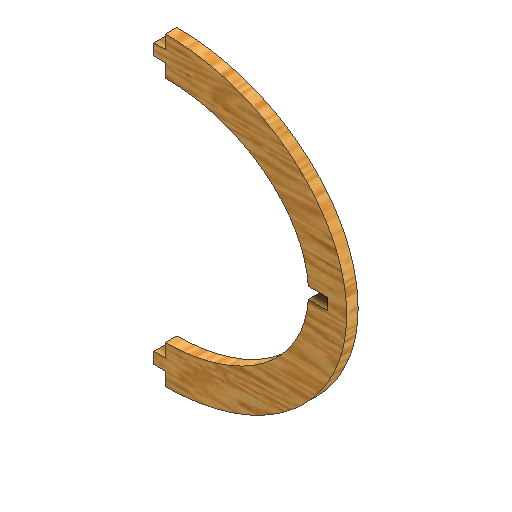
# Autodesk Inventor part: Arch Rear Outer
Saved by Autodesk Inventor 2025.2 (Build 292293000, 293)
## iProperties
Created: 2025-01-15
Part Number: Arch Rear Outer
Material: Plywood, Sheathing
Document SubType Name: Modeling
Designer: alexb
Density: 0.552 g/cm^3
Appearance: Plywood - New
Author: alexb
Autodesk Inventor part; units mm, degrees
ref_plane "YZ Plane" through (0, 0, 0) normal (1, 0, 0) x (0, 1, 0)
ref_plane "XZ Plane" through (0, 0, 0) normal (0, 1, 0) x (-1, 0, 0)
ref_plane "XY Plane" through (0, 0, 0) normal (0, 0, 1) x (1, 0, 0)
sketch "Sketch1" plane through (0, 0, 0) normal (0, 0, 1) x (1, 0, 0)
  ellipse E0 centre (0, 0) end of major axis (95, 0) minor radius 80 (0, -80) -> (0, 80) ccw
  ellipse E1 centre (0, 0) end of major axis (75, 0) minor radius 60 (0, -60) -> (0, 60) ccw
  line L0 (0, 80) -> (0, 73)
  line L1 (0, 73) -> (-6, 73)
  line L2 (-6, 73) -> (-6, 67)
  line L3 (-6, 67) -> (0, 67)
  line L4 (0, 67) -> (0, 60)
  line L5 (75, 0) -> (95, 0) construction
  line L6 (0, -73) -> (-6, -73)
  line L7 (-6, -73) -> (-6, -67)
  line L8 (-6, -67) -> (0, -67)
  line L9 (0, -60) -> (0, -67)
  line L10 (0, -73) -> (0, -80)
  line L11 (85, -35.7275) -> (85, 35.7275) construction
  line L12 (85, 3) -> (85, -3)
  line L13 (85, 3) -> (74.9062, 3)
  line L14 (85, -3) -> (74.9062, -3)
  point P0 (85, 0)
  dimension "d0" = 80
  dimension "d2" = 75
  dimension "d3" = 60
  dimension "d4" = 95
  dimension "d6" = 6
  dimension "d7" = 6
  constraints: 30 end point, 7 vertical, 5 perpendicular, 4 symmetric about line, 3 horizontal, 3 midpoint, 2 coincident, 2 equal length, 1 point on line, 13 other
  measures "d6" distance of L1.end L2.end
  measures "d7" distance between parallel lines of L14 L13
extrude "Extrusion1" add sketch "Sketch1" along normal blind 6 contours L10 L6 L7 L8 L9 E1 L14 L12 L13 L4 L3 L2 L1 L0 E0
body "Solid1"
